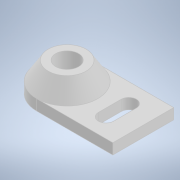
# Autodesk Inventor part: Coupler for Section
Saved by Autodesk Inventor 2022 (Build 260153000, 153)
## iProperties
Created: 2022-03-17
Part Number: Coupler for Section
Material: Generic
Document SubType Name: Modeling
Designer: Harsh Chopra
Density: 1 g/cm^3
Appearance: Default
Author: Harsh Chopra
Autodesk Inventor part; units mm, degrees
ref_plane "YZ Plane" through (0, 0, 0) normal (1, 0, 0) x (0, 1, 0)
ref_plane "XZ Plane" through (0, 0, 0) normal (0, 1, 0) x (-1, 0, 0)
sketch "Sketch1" plane through (0, 0, 0) normal (0, 1, 0) x (-1, 0, 0)
  line L0 (31.75, 25.4) -> (-31.75, 25.4)
  line L1 (-31.75, 25.4) -> (-31.75, -25.4)
  line L2 (-31.75, -25.4) -> (31.75, -25.4)
  line L3 (31.75, -25.4) -> (31.75, 25.4)
  line L4 (31.75, 25.4) -> (-31.75, -25.4) construction
  line L5 (-31.75, 25.4) -> (31.75, -25.4) construction
  arc A0 (31.75, -25.4) -> (31.75, 25.4) centre (31.75, 0) ccw
  point P0 (0, 0)
  dimension "d5" = 63.5
  dimension "d6" = 50.8
  constraints: 12 end point, 3 midpoint, 2 parallel, 2 point on circle, 1 centre point, 1 horizontal, 1 perpendicular
  measures "d5" distance of L2.end L1.end
  measures "d6" distance of L1.end L0.end
extrude "Extrusion1" add sketch "Sketch1" against normal blind 8.89
sketch "Sketch2" plane through (0, 0, 0) normal (0, 1, 0) x (1, 0, 0)
  line L0 (31.75, -25.4) -> (31.75, 25.4) projected
  line L1 (-31.75, -25.4) -> (31.75, -25.4) projected
  line L2 (31.75, 25.4) -> (-31.75, 25.4) projected
  arc A0 (-31.75, 25.4) -> (-31.75, -25.4) centre (-31.75, 0) ccw projected
  line L3 (31.75, 0) -> (16.51, 0)
  line L4 (3.81, -9.525) -> (16.51, -9.525)
  line L5 (16.51, -9.525) -> (16.51, 9.525)
  line L6 (16.51, 9.525) -> (3.81, 9.525)
  line L7 (3.81, 9.525) -> (3.81, -9.525)
  line L8 (3.81, -9.525) -> (16.51, 9.525) construction
  line L9 (16.51, -9.525) -> (3.81, 9.525) construction
  arc A1 (3.81, -9.525) -> (16.51, -9.525) centre (10.16, -9.525) ccw
  arc A2 (16.51, 9.525) -> (3.81, 9.525) centre (10.16, 9.525) ccw
  point P0 (0, 0)
  dimension "d9" = 15.24
  dimension "d10" = 12.7
  dimension "d11" = 19.05
  constraints: 14 end point, 4 midpoint, 4 point on circle, 2 centre point, 2 horizontal, 2 parallel, 1 perpendicular
  measures "d9" distance of L3.start L3.end
  measures "d10" distance of L5.end L6.end
  measures "d11" distance of L4.end L5.end
extrude "Extrusion2" cut sketch "Sketch2" against normal blind 8.89 contours L5 L4 L7 L6 | A1 L4 | L6 A2
sketch "Sketch3" plane through (0, 0, 0) normal (0, 1, 0) x (1, 0, 0)
  arc A0 (-31.75, 25.4) -> (-31.75, -25.4) centre (-31.75, 0) ccw projected
  circle A1 centre (-31.75, 0) radius 25.4
  point P0 (0, 0)
  dimension "d14" = 50.8
  constraints: 1 centre point, 1 coincident
  measures "d14" diameter of A1
ref_plane "Work Plane1" through (0, 15.24, 0) normal (0, 1, 0) x (1, 0, 0)
sketch "Sketch5" plane through (0, 15.24, 0) normal (0, 1, 0) x (1, 0, 0)
  arc A0 (-31.75, 25.4) -> (-31.75, -25.4) centre (-31.75, 0) ccw projected
  circle A1 centre (-31.75, 0) radius 15.875
  point P0 (0, 0)
  dimension "d20" = 31.75
  constraints: 1 centre point, 1 coincident
  measures "d20" diameter of A1
loft "Loft1" add profiles "Sketch3", "Sketch5"
sketch "Sketch6" plane through (-31.75, 15.24, 0) normal (0, 1, 0) x (1, 0, 0)
  circle A0 centre (0, 0) radius 15.875 projected
  circle A1 centre (0, 0) radius 9.525
  point P0 (31.75, 0)
  dimension "d25" = 19.05
  constraints: 1 centre point, 1 coincident
  measures "d25" diameter of A1
extrude "Extrusion3" cut sketch "Sketch6" against normal blind 50.8 contours A1
body "Solid1"
